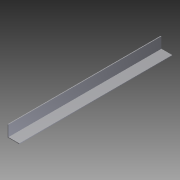
# Autodesk Inventor part: 8 ball top L frame
Saved by Autodesk Inventor 2012 (Build 160160000, 160)
## iProperties
Created: 2013-10-29
Part Number: 8 ball top L frame
Material: Default
Document SubType Name: Modeling
Designer: Bryce
Density: 1 g/cm^3
Author: Bryce
Autodesk Inventor part; units mm, degrees
ref_plane "YZ Plane" through (0, 0, 0) normal (1, 0, 0) x (0, 1, 0)
ref_plane "XZ Plane" through (0, 0, 0) normal (0, 1, 0) x (-1, 0, 0)
ref_plane "XY Plane" through (0, 0, 0) normal (0, 0, 1) x (1, 0, 0)
sketch "Sketch1" plane through (0, 0, 0) normal (0, 0, 1) x (1, 0, 0)
  line L0 (0, 0) -> (25.4, 0)
  line L1 (25.4, 0) -> (25.4, 1.5875)
  line L2 (1.5875, 25.4) -> (0, 25.4)
  line L3 (0, 25.4) -> (0, 0)
  line L4 (1.5875, 25.4) -> (1.5875, 1.5875)
  line L5 (1.5875, 1.5875) -> (25.4, 1.5875)
  dimension "d0" = 1.5875
  dimension "d1" = 1.5875
  dimension "d2" = 25.4
  dimension "d3" = 25.4
  constraints: 12 end point, 2 parallel, 1 horizontal, 1 perpendicular
  measures "d0" distance between parallel lines of L4 L3
  measures "d1" distance between parallel lines of L0 L5
  measures "d2" distance of L0.start L0.end
  measures "d3" distance of L2.end L0.start
extrude "Extrusion1" add sketch "Sketch1" along normal blind 334.9625
equation "\"d0\" = d1"
equation "\"d2\" = d3"
body "Solid1"
